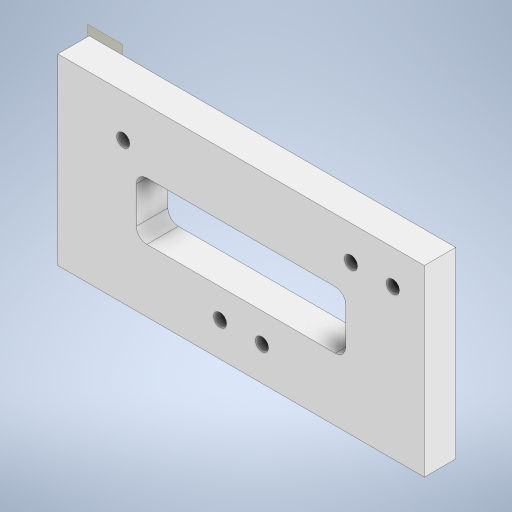
# Autodesk Inventor part: 61
Saved by Autodesk Inventor 2024.3 (Build 283343000, 343)
## iProperties
Created: 2024-09-08
Part Number: 61
Material: 아크릴, 선명
Document SubType Name: Modeling
Designer: 구지현
Density: 1.19 g/cm^3
Appearance: 흰색
Author: 구지현
Autodesk Inventor part; units mm, degrees
ref_plane "YZ Plane" through (0, 0, 0) normal (1, 0, 0) x (0, 1, 0)
ref_plane "XZ Plane" through (0, 0, 0) normal (0, 1, 0) x (-1, 0, 0)
ref_plane "XY Plane" through (0, 0, 0) normal (0, 0, 1) x (1, 0, 0)
ref_plane "작업 평면1" through (0, 0, 0) normal (0, 0, 1) x (1, 0, 0)
sketch "스케치1" plane through (0, 0, 0) normal (0, 0, 1) x (1, 0, 0)
  line L0 (0, 0) -> (6, 0) projected
  line L1 (6, 0) -> (6, 35) projected
  line L2 (0, 35) -> (6, 35) projected
  line L3 (0, 0) -> (0, 35) projected
  line L4 (0, 35) -> (70, 35)
  line L5 (70, 35) -> (70, 0)
  line L6 (70, 0) -> (0, 0)
  line L7 (0, 0) -> (0, 35)
  dimension "d4" = 0
  dimension "d0" = 70
  constraints: 8 end point, 2 parallel, 1 horizontal, 1 perpendicular
  measures "d0" distance of L5.end L6.end
extrude "돌출1" add sketch "스케치1" along normal blind 6
sketch "스케치2" plane through (0, 0, 6) normal (0, 0, 1) x (1, 0, 0)
  circle A0 centre (39, 6.5) radius 1.25 projected
  circle A1 centre (31, 6.5) radius 1.25 projected
  line L0 (25, 3) -> (45, 3) projected
  line L1 (45, 3) -> (45, 10) projected
  line L2 (45, 10) -> (25, 10) projected
  line L3 (25, 10) -> (25, 3) projected
  point P0 (0, 0)
extrude "돌출2" cut sketch "스케치2" against normal blind 6 contours A0 | A1
sketch "스케치3" plane through (0, 0, 6) normal (0, 0, 1) x (1, 0, 0)
  circle A0 centre (56, 28.5) radius 1.25 projected
  circle A1 centre (64, 28.5) radius 1.25 projected
  circle A2 centre (56, 28.5) radius 1.25 projected
  line L0 (50, 32) -> (70, 32) projected
  line L1 (70, 32) -> (70, 25) projected
  line L2 (70, 25) -> (50, 25) projected
  line L3 (50, 25) -> (50, 32) projected
  circle A3 centre (12.5, 27) radius 1.25 projected
  line L4 (9, 32) -> (16, 32) projected
  line L5 (16, 22) -> (16, 32) projected
  line L6 (9, 22) -> (16, 22) projected
  line L7 (9, 32) -> (9, 22) projected
  point P0 (0, 0)
extrude "돌출3" cut sketch "스케치3" against normal blind 6 contours A0 | A1 | A3
sketch "스케치4" plane through (0, 0, 6) normal (0, 0, 1) x (1, 0, 0)
  line L0 (15, 14) -> (15, 21) projected
  arc A0 (17, 23) -> (15, 21) centre (17, 21) ccw projected
  line L1 (17, 23) -> (53, 23) projected
  arc A1 (55, 21) -> (53, 23) centre (53, 21) ccw projected
  line L2 (55, 21) -> (55, 14) projected
  arc A2 (53, 12) -> (55, 14) centre (53, 14) ccw projected
  line L3 (53, 12) -> (17, 12) projected
  arc A3 (15, 14) -> (17, 12) centre (17, 14) ccw projected
  circle A4 centre (64, 28.5) radius 1.25 projected
  circle A5 centre (56, 28.5) radius 1.25 projected
  circle A6 centre (14, 27) radius 1.25 projected
  circle A7 centre (39, 6.5) radius 1.25 projected
  circle A8 centre (31, 6.5) radius 1.25 projected
  line L4 (0, 0) -> (70, 0) projected
  line L5 (70, 0) -> (70, 35) projected
  line L6 (70, 35) -> (0, 35) projected
  line L7 (0, 35) -> (0, 0) projected
  point P0 (0, 0)
extrude "돌출4" cut sketch "스케치4" against normal blind 6 contours L0 A0 L1 A1 L2 A2 L3 A3
